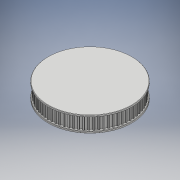
# Autodesk Inventor part: Gear 70 Teeth
Saved by Autodesk Inventor 2018 (Build 220112000, 112)
## iProperties
Created: 2018-05-29
Part Number: Gear 70 Teeth
Material: Generic
Document SubType Name: Modeling
Designer: P301319
Density: 1 g/cm^3
Appearance: Default
Author: P301319
Autodesk Inventor part; units mm, degrees
ref_plane "YZ Plane" through (0, 0, 0) normal (1, 0, 0) x (0, 1, 0)
ref_plane "XZ Plane" through (0, 0, 0) normal (0, 1, 0) x (-1, 0, 0)
ref_plane "XY Plane" through (0, 0, 0) normal (0, 0, 1) x (1, 0, 0)
sketch "Tooth" plane through (0, 0, 0) normal (0, 0, 1) x (1, 0, 0)
  arc A0 (0, 33.4225) -> (-1.4995, 33.3889) centre (0, 0) ccw construction
  line L0 (0, 0) -> (0, 33.4225) construction
  line L1 (0, 0) -> (-1.4995, 33.3889) construction
  circle A1 centre (0, 0) radius 32.2825 construction
  arc A2 (-0.7704, 32.7733) -> (0, 32.2825) centre (0, 33.1325) ccw
  arc A3 (0.61, 33.417) -> (0, 33.4225) centre (0, 0) ccw construction
  arc A4 (-0.8961, 33.1901) -> (-0.7704, 32.7733) centre (0.61, 33.417) ccw
  arc A5 (-1.1519, 33.4027) -> (-1.4995, 33.3889) centre (0, 0) ccw
  arc A6 (-0.8961, 33.1901) -> (-1.1519, 33.4027) centre (-1.1433, 33.1528) ccw
  arc A7 (0, 32.2825) -> (0.7704, 32.7733) centre (0, 33.1325) ccw
  arc A8 (0.7704, 32.7733) -> (0.8961, 33.1901) centre (-0.61, 33.417) ccw
  arc A9 (1.4995, 33.3889) -> (1.1519, 33.4027) centre (0, 0) ccw
  arc A10 (1.1519, 33.4027) -> (0.8961, 33.1901) centre (1.1433, 33.1528) ccw
  arc A11 (1.5892, 35.3869) -> (-1.5892, 35.3869) centre (0, 0) ccw
  line L2 (1.4995, 33.3889) -> (1.5892, 35.3869)
  line L3 (-1.4995, 33.3889) -> (-1.5892, 35.3869)
  dimension "d2" = 33.4225
  dimension "d3" = 1.5
  dimension "d4" = 1.14
  dimension "d5" = 0.85
  dimension "d6" = 0.61
  dimension "d7" = 0.25
  dimension "d8" = 2
  constraints: 22 point on circle, 11 centre point, 8 end point, 6 symmetric about line, 5 coincident, 4 line through centre, 3 tangent, 2 vertical alignment, 1 concentric, 1 vertical, 7 other
  measures "d2" radius of A0
  measures "d5" radius of A2
  measures "d7" radius of A6
  measures "d8" radial gap between concentric circles of A11 A0
sketch "Sketch2" plane through (0, 0, 0) normal (0, 0, 1) x (1, 0, 0)
  circle A0 centre (0, 0) radius 33.4225
  arc A1 (-1.1519, 33.4027) -> (-1.4995, 33.3889) centre (0, 0) ccw projected
  arc A2 (1.4995, 33.3889) -> (1.1519, 33.4027) centre (0, 0) ccw projected
  dimension "Radius" = 33.4225
  constraints: 1 centre point, 1 coincident
  measures "Radius" radius of A0
extrude "Gear Solid Extrusion" add sketch "Sketch2" along normal blind 10
extrude "Tooth Cut-Out Extrusion" cut sketch "Tooth" along normal blind 10
pattern_circular "Teeth Array" count 70 over 360 about axis through (0, 0, 0) along (0, 0, 1) of "Tooth Cut-Out Extrusion"
sketch "Sketch3" plane through (0, 0, 10) normal (0, 0, 1) x (1, 0, 0)
  circle A0 centre (0, 0) radius 34.4225
  dimension "d17" = 34.4225
  constraints: 1 centre point, 1 coincident
  measures "d17" radius of A0
extrude "Flange Extrusion Front" add sketch "Sketch3" along normal blind 1.5
sketch "Sketch4" plane through (0, 0, 0) normal (0, 0, -1) x (-1, 0, 0)
  circle A0 centre (0, 0) radius 34.4225
  dimension "d20" = 34.4225
  constraints: 1 centre point, 1 coincident
  measures "d20" radius of A0
extrude "Flange Extrusion Back" add sketch "Sketch4" along normal blind 1.5
fillet "Flange Fillet" radius 0.25 4 edges at (34.4225, 0, -1.5) (-34.4225, 0, 11.5) (-34.4225, 0, 10) (34.4225, 0, 0)
equation "\"d3\" = HalfPitch"
equation "\"d12\" = ToothWidth"
equation "\"d21\" = FlangeWidth"
equation "\"HalfPitch\" = 1.5"
equation "\"ToothWidth\" = 10"
equation "\"FlangeWidth\" = 1.5"
body "Solid1"
